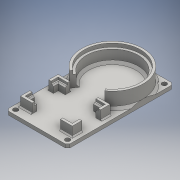
# Autodesk Inventor part: main-base
Saved by Autodesk Inventor 2016 (Build 200138000, 138)
## iProperties
Created: 2016-12-19
Part Number: main-base
Material: Generic
Document SubType Name: Modeling
Designer: Matt Ruffner
Density: 1 g/cm^3
Appearance: Default
Author: Matt Ruffner
Autodesk Inventor part; units mm, degrees
ref_plane "YZ Plane" through (0, 0, 0) normal (1, 0, 0) x (0, 1, 0)
ref_plane "XZ Plane" through (0, 0, 0) normal (0, 1, 0) x (-1, 0, 0)
ref_plane "XY Plane" through (0, 0, 0) normal (0, 0, 1) x (1, 0, 0)
sketch "Sketch2" plane through (0, 0, 0) normal (0, 0, 1) x (1, 0, 0)
  line L0 (-5.2343, 1.013) -> (42.7657, 1.013)
  line L1 (44.7657, -0.987) -> (44.7657, -86.987)
  line L2 (42.7657, -88.987) -> (-5.2343, -88.987)
  line L3 (-7.2343, -86.987) -> (-7.2343, -0.987)
  circle A0 centre (-3.2343, -2.987) radius 2
  circle A1 centre (40.7657, -2.987) radius 2
  circle A2 centre (40.7657, -84.987) radius 2
  circle A3 centre (-3.2343, -84.987) radius 2
  line L4 (-5.2343, 1.013) -> (-7.2343, -0.987)
  line L5 (42.7657, 1.013) -> (44.7657, -0.987)
  line L6 (42.7657, -88.987) -> (44.7657, -86.987)
  line L7 (-7.2343, -86.987) -> (-5.2343, -88.987)
  point P0 (0, 0)
  point P1 (-7.2343, 1.013)
  point P2 (44.7657, -88.987)
  point P3 (44.7657, 1.013)
  point P4 (-7.2343, -88.987)
  dimension "d0" = 52
  dimension "d1" = 90
  dimension "d2" = 4
  dimension "d3" = 4
  dimension "d4" = 4
  dimension "d5" = 4
  dimension "d6" = 4
  dimension "d7" = 4
  dimension "d8" = 4
  dimension "d9" = 4
  dimension "d10" = 4
  dimension "d11" = 4
  dimension "d12" = 4
  dimension "d13" = 4
  dimension "d14" = 2
  dimension "d15" = 2
  dimension "d16" = 2
  dimension "d17" = 2
  dimension "d18" = 2
  dimension "d19" = 2
  dimension "d20" = 2
  dimension "d21" = 2
  constraints: 16 end point, 8 point on line, 4 centre point, 2 parallel, 1 horizontal, 1 perpendicular
  measures "d0" distance of point (44.766, -88.987) point (-7.234, -88.987)
  measures "d1" distance of point (44.766, 1.013) point (44.766, -88.987)
  measures "d2" diameter of A0
  measures "d3" diameter of A1
  measures "d4" diameter of A3
  measures "d5" diameter of A2
  measures "d6" distance from line of L2 A3.centre
  measures "d7" distance from line of L3 A3.centre
  measures "d8" distance from line of L2 A2.centre
  measures "d9" distance from line of L1 A2.centre
  measures "d10" distance from line of L1 A1.centre
  measures "d11" distance from line of L0 A1.centre
  measures "d12" distance from line of L3 A0.centre
  measures "d13" distance from line of L0 A0.centre
  measures "d14" distance of L0.start point (-7.234, 1.013)
  measures "d15" distance of L3.end point (-7.234, 1.013)
  measures "d16" distance of L0.end point (44.766, 1.013)
  measures "d17" distance of L1.start point (44.766, 1.013)
  measures "d18" distance of L2.start point (44.766, -88.987)
  measures "d19" distance of L1.end point (44.766, -88.987)
  measures "d20" distance of L3.start point (-7.234, -88.987)
  measures "d21" distance of L2.end point (-7.234, -88.987)
extrude "Extrusion1" add sketch "Sketch2" along normal blind 3
sketch "Sketch3" plane through (0, 0, 3) normal (0, 0, 1) x (1, 0, 0)
  arc A0 (31.3844, -43.0083) -> (6.1471, -43.0083) centre (18.7657, -24.987) ccw
  line L0 (-7.2343, -0.987) -> (-7.2343, -86.987) projected
  line L1 (42.7657, 1.013) -> (-5.2343, 1.013) projected
  arc A1 (32.5316, -44.6466) -> (4.9999, -44.6466) centre (18.7657, -24.987) ccw
  line L2 (6.1471, -43.0083) -> (4.9999, -44.6466)
  line L3 (18.7657, -24.987) -> (62.8493, -24.987) construction
  line L4 (31.3844, -43.0083) -> (32.5316, -44.6466)
  line L5 (18.7657, -24.987) -> (69.9782, -24.987) construction
  point P0 (0, 0)
  dimension "d24" = 44
  dimension "d25" = 26
  dimension "d26" = 26
  dimension "d27" = 48
  dimension "d28" = 125
  dimension "d29" = 55
  constraints: 8 end point, 4 point on circle, 2 centre point, 2 horizontal, 1 coincident
  measures "d24" diameter of A0
  measures "d25" distance from line of L0 A0.centre
  measures "d26" distance from line of L1 A0.centre
  measures "d27" diameter of A1
  measures "d28" angle of L2 L3
  measures "d29" angle of L4 L5
extrude "Extrusion2" add sketch "Sketch3" along normal blind 10
sketch "Sketch4" plane through (0, 0, 3) normal (0, 0, 1) x (1, 0, 0)
  arc A0 (31.3844, -43.0083) -> (6.1471, -43.0083) centre (18.7657, -24.987) ccw projected
  arc A1 (32.5316, -44.6466) -> (4.9999, -44.6466) centre (18.7657, -24.987) ccw projected
  arc A2 (33.6787, -46.2849) -> (3.8528, -46.2849) centre (18.7657, -24.987) ccw
  line L0 (6.1471, -43.0083) -> (3.8528, -46.2849)
  line L1 (6.1471, -43.0083) -> (4.9999, -44.6466) projected
  line L2 (31.3844, -43.0083) -> (33.6787, -46.2849)
  arc A3 (32.5316, -44.6466) -> (4.9999, -44.6466) centre (18.7657, -24.987) ccw
  point P0 (0, 0)
  constraints: 6 point on circle, 5 end point, 2 centre point, 2 coincident, 1 collinear, 1 midpoint
extrude "Extrusion3" add sketch "Sketch4" along normal blind 13 contours A1 L0 A2 L2
chamfer "Chamfer1" distance 2 angle 45 1 edges at (18.7657, -2.987, 3)
chamfer "Chamfer2" distance 2 angle 45 4 edges at (37.1505, -6.6022, 3) (0.381, -6.6022, 3) (41.828, -36.9924, 3) (-4.2965, -36.9924, 3)
ref_plane "Work Plane2" through (0, 0, 6.25) normal (0, 0, 1) x (1, 0, 0)
sketch "Sketch5" plane through (0, 0, 6.25) normal (0, 0, 1) x (1, 0, 0)
  circle A0 centre (-3.2343, -2.987) radius 2 projected
  circle A1 centre (40.7657, -2.987) radius 2 projected
  circle A2 centre (-3.2343, -2.987) radius 4
  circle A3 centre (40.7657, -2.987) radius 4
  point P0 (0, 0)
  point P1 (-1.4896, -5.6551)
  point P2 (-0.5661, -4.7316)
  point P3 (38.0976, -4.7316)
  point P4 (39.0211, -5.6551)
  dimension "d41" = 8
  dimension "d42" = 8
  constraints: 2 centre point, 2 coincident, 2 other
  measures "d41" diameter of A2
  measures "d42" diameter of A3
extrude "Extrusion4" cut sketch "Sketch5" against normal up to surface (3.25 mm away) contours A0 | A1 | A2 | A3
sketch "Sketch10" plane through (0, 0, 3) normal (0, 0, 1) x (1, 0, 0)
  line L0 (-7.2343, -35.3793) -> (-7.2343, -86.987) projected
  line L1 (-5.2343, -88.987) -> (42.7657, -88.987) projected
  line L2 (-5.2343, -58.987) -> (42.0131, -58.987)
  line L3 (42.0131, -58.987) -> (42.0131, -70.987)
  line L4 (42.0131, -70.987) -> (-5.2343, -70.987)
  line L5 (-5.2343, -70.987) -> (-5.2343, -58.987)
  line L6 (6.7657, -47.2465) -> (30.7657, -47.2465)
  line L7 (30.7657, -47.2465) -> (30.7657, -83.163)
  line L8 (30.7657, -83.163) -> (6.7657, -83.163)
  line L9 (6.7657, -83.163) -> (6.7657, -47.2465)
  line L10 (-3.2343, -80.987) -> (-3.2343, -70.987)
  line L11 (-3.2343, -58.987) -> (-3.2343, -48.987)
  line L12 (-1.2343, -78.987) -> (-1.2343, -70.987)
  line L13 (-1.2343, -58.987) -> (-1.2343, -50.987)
  line L14 (38.7657, -78.987) -> (30.7657, -78.987)
  line L15 (6.7657, -78.987) -> (-1.2343, -78.987)
  line L16 (40.7657, -80.987) -> (30.7657, -80.987)
  line L17 (6.7657, -80.987) -> (-3.2343, -80.987)
  line L18 (38.7657, -50.987) -> (38.7657, -58.987)
  line L19 (38.7657, -70.987) -> (38.7657, -78.987)
  line L20 (40.7657, -48.987) -> (40.7657, -58.987)
  line L21 (40.7657, -70.987) -> (40.7657, -80.987)
  line L22 (-3.2343, -48.987) -> (6.7657, -48.987)
  line L23 (30.7657, -48.987) -> (40.7657, -48.987)
  line L24 (-1.2343, -50.987) -> (6.7657, -50.987)
  line L25 (30.7657, -50.987) -> (38.7657, -50.987)
  point P0 (0, 0)
  dimension "d64" = 40
  dimension "d65" = 28
  constraints: 48 end point, 20 parallel, 16 point on line, 10 perpendicular, 6 horizontal
  measures "d64" distance of L14.start L12.start
  measures "d65" distance of L18.start L14.start
extrude "Extrusion7" add sketch "Sketch10" along normal blind 8 contours L11 L22 L9 L24 L13 L2 | L4 L12 L15 L9 L17 L10 | L18 L25 L7 L23 L20 L2 | L4 L21 L16 L7 L14 L19
sketch "Sketch11" plane through (0, 0, 3) normal (0, 0, 1) x (1, 0, 0)
  line L0 (-3.2343, -58.987) -> (-1.2343, -58.987) projected
  line L1 (38.7657, -50.987) -> (38.7657, -58.987) projected
  line L2 (6.7657, -80.987) -> (6.7657, -78.987) projected
  line L3 (-1.2343, -50.987) -> (6.7657, -50.987) projected
  line L4 (-1.2343, -78.987) -> (-1.2343, -70.987) projected
  line L5 (38.7657, -78.987) -> (30.7657, -78.987) projected
  line L6 (30.7657, -50.987) -> (30.7657, -48.987) projected
  line L7 (6.7657, -78.987) -> (-1.2343, -78.987) projected
  line L8 (38.7657, -70.987) -> (38.7657, -78.987) projected
  line L9 (30.7657, -50.987) -> (38.7657, -50.987) projected
  line L10 (-1.2343, -58.987) -> (-1.2343, -50.987) projected
  line L11 (-1.2343, -58.987) -> (0.7657, -58.987)
  line L12 (36.7657, -58.987) -> (38.7657, -58.987)
  line L13 (6.7657, -78.987) -> (6.7657, -76.987)
  line L14 (6.7657, -52.987) -> (6.7657, -50.987)
  line L15 (38.7659, -70.987) -> (36.7657, -70.987)
  line L16 (0.7657, -70.987) -> (-1.2343, -70.987)
  line L17 (30.7657, -78.987) -> (30.7657, -76.987)
  line L18 (30.7657, -52.987) -> (30.7657, -50.987)
  line L19 (0.7657, -52.987) -> (6.7657, -52.987)
  line L20 (30.7657, -52.987) -> (36.7657, -52.987)
  line L21 (36.7657, -52.987) -> (36.7657, -58.987)
  line L22 (36.7657, -70.987) -> (36.7657, -76.987)
  line L23 (36.7657, -76.987) -> (30.7657, -76.987)
  line L24 (6.7657, -76.987) -> (0.7657, -76.987)
  line L25 (0.7657, -76.987) -> (0.7657, -70.987)
  line L26 (0.7657, -58.987) -> (0.7657, -52.987)
  line L27 (38.7657, -70.987) -> (36.7657, -70.987)
  point P0 (0, 0)
  constraints: 34 end point, 8 parallel, 7 horizontal, 4 perpendicular, 4 vertical
extrude "Extrusion8" add sketch "Sketch11" along normal blind 6
chamfer "Chamfer3" distance 1 angle 45 15 edges at (0.7657, -55.987, 9) (3.7657, -52.987, 9) (0.7657, -73.987, 9) (6.7657, -77.987, 9) (33.7657, -52.987, 9) (36.7657, -55.987, 9) (36.7657, -73.987, 9) (33.7657, -76.987, 9) (1.7657, -48.987, 3) (-3.2343, -53.987, 3) (-3.2343, -75.987, 3) (40.7657, -53.987, 3) (40.7657, -75.987, 3) (35.7657, -80.987, 3) (1.7657, -80.987, 3)
sketch "Sketch12" plane through (0, 0, 11) normal (0, 0, 1) x (1, 0, 0)
  line L0 (-4.2343, -47.987) -> (-4.2343, -58.987) projected
  line L1 (-4.2343, -70.987) -> (-4.2343, -81.987) projected
  line L2 (41.7657, -81.987) -> (41.7657, -70.987) projected
  line L3 (41.7657, -58.987) -> (41.7657, -48.987) projected
  line L4 (-4.2343, -56.987) -> (41.7657, -56.987)
  line L5 (41.7657, -56.987) -> (41.7657, -72.987)
  line L6 (41.7657, -72.987) -> (-4.2343, -72.987)
  line L7 (-4.2343, -72.987) -> (-4.2343, -56.987)
  line L8 (-3.2343, -58.987) -> (-1.2343, -58.987) projected
  line L9 (-1.2343, -70.987) -> (-3.2343, -70.987) projected
  point P0 (0, 0)
  dimension "d87" = 2
  dimension "d88" = 2
  constraints: 8 end point, 2 parallel, 2 point on line, 1 horizontal, 1 perpendicular
  measures "d87" distance between parallel lines of L4 L8
  measures "d88" distance between parallel lines of L9 L6
extrude "Extrusion9" cut sketch "Sketch12" against normal up to surface (8 mm away)
chamfer "Chamfer4" distance 1 angle 45 1 edges at (2.7657, -76.987, 9)
equation "\"d15\" = d14"
equation "\"d17\" = d16"
equation "\"d18\" = d16"
equation "\"d19\" = d18"
equation "\"d20\" = d16"
equation "\"d21\" = d20"
body "Solid1"
